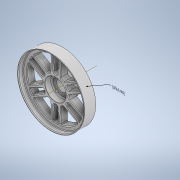
# Autodesk Inventor part: RPF1s
Saved by Autodesk Inventor 2020 (Build 240168000, 168)
## iProperties
Created: 2022-01-06
Part Number: RPF1s
Material: Generic
Document SubType Name: Modeling
Designer: harry
Density: 1 g/cm^3
Appearance: Default
Author: harry
Autodesk Inventor part; units mm, degrees
ref_plane "YZ Plane" through (0, 0, 0) normal (1, 0, 0) x (0, 1, 0)
ref_plane "XZ Plane" through (0, 0, 0) normal (0, 1, 0) x (-1, 0, 0)
ref_plane "Work Plane1" through (0, 0, 35) normal (0, 0, 1) x (1, 0, 0)
sketch "Sketch2" plane through (0, 0, 35) normal (0, 0, 1) x (1, 0, 0)
  circle A0 centre (0, 0) radius 75.361
  circle A1 centre (0, 0) radius 37.761
  circle A2 centre (-57.1499, 18.5691) radius 7.75
  circle A3 centre (0, 60.091) radius 7.75
  circle A4 centre (57.1499, 18.5691) radius 7.75
  circle A5 centre (35.3206, -48.6146) radius 7.75
  circle A6 centre (-35.3206, -48.6146) radius 7.75
  dimension "d2" = 37.6
  dimension "d3" = 150.722
  dimension "d4" = 15.5
  dimension "d7" = 360
  dimension "d11" = 60.091
  constraints: 7 centre point, 4 coincident, 1 vertical alignment, 14 other
  measures "d2" radial gap between concentric circles of A0 A1
  measures "d3" diameter of A0
  measures "d4" diameter of A2
  measures "d11" distance of A0.centre A3.centre
sketch "Sketch3" plane through (0, 0, 0) normal (1, 0, 0) x (0, 1, 0)
  line L0 (-273.6168, 35) -> (133.524, 35) construction
  line L1 (75.361, 35) -> (75.361, 71.76) construction
  line L2 (75.361, 35) -> (-75.361, 35) construction
  line L3 (75.361, 71.76) -> (75.361, 35)
  line L4 (0, -28.552) -> (0, 171.312) construction
  line L5 (75.361, 71.76) -> (0, 71.76)
  line L6 (0, 35) -> (0, 71.76)
  line L7 (0, 35) -> (75.361, 35)
  point P0 (0, 0)
  dimension "d91" = 36.76
  constraints: 10 end point, 2 collinear, 2 perpendicular, 2 point on line, 1 midpoint
  measures "d91" distance between parallel lines of L2 L5
revolve "Revolution1" add sketch "Sketch3" angle 360 about axis through (0, 0, -10) along (0, 0, 1)
extrude "Extrusion1" cut sketch "Sketch2" along normal through all contours A1 | A2 | A3 | A4 | A5 | A6
ref_plane "Work Plane2" through (0, 0, 71.76) normal (0, 0, 1) x (1, 0, 0)
sketch "Sketch4" plane through (0, 0, 71.76) normal (0, 0, 1) x (1, 0, 0)
  line L0 (-13, 95.7863) -> (-17, 184.2173)
  line L1 (-34.3721, 75.9448) -> (-32.5, 182.1229)
  circle A0 centre (0, 0) radius 185
  line L2 (13, 95.7863) -> (17, 184.2173)
  line L3 (34.3721, 75.9448) -> (32.5, 182.1229)
  arc A1 (-13, 95.7863) -> (13, 95.7863) centre (0, 96.3743) ccw
  circle A2 centre (0, 0) radius 68.5449
  circle A3 centre (0, 0) radius 83.361
  circle A4 centre (0, 0) radius 68.5449
  arc A5 (-89.4533, 36.6348) -> (-76.4533, 59.1515) centre (-83.4626, 48.1871) ccw
  line L4 (-48.5841, 67.7395) -> (-141.4731, 119.2073)
  line L5 (-76.4533, 59.1515) -> (-151.0368, 106.8311)
  line L6 (-89.4533, 36.6348) -> (-168.0368, 77.3862)
  line L7 (-82.9562, 8.2053) -> (-173.9731, 62.9156)
  arc A6 (-76.4533, -59.1515) -> (-89.4533, -36.6348) centre (-83.4626, -48.1871) ccw
  line L8 (-82.9562, -8.2053) -> (-173.9731, -62.9156)
  line L9 (-89.4533, -36.6348) -> (-168.0368, -77.3862)
  line L10 (-76.4533, -59.1515) -> (-151.0368, -106.8311)
  line L11 (-48.5841, -67.7395) -> (-141.4731, -119.2073)
  arc A7 (13, -95.7863) -> (-13, -95.7863) centre (0, -96.3743) ccw
  line L12 (-34.3721, -75.9448) -> (-32.5, -182.1229)
  line L13 (-13, -95.7863) -> (-17, -184.2173)
  line L14 (13, -95.7863) -> (17, -184.2173)
  line L15 (34.3721, -75.9448) -> (32.5, -182.1229)
  arc A8 (89.4533, -36.6348) -> (76.4533, -59.1515) centre (83.4626, -48.1871) ccw
  line L16 (48.5841, -67.7395) -> (141.4731, -119.2073)
  line L17 (76.4533, -59.1515) -> (151.0368, -106.8311)
  line L18 (89.4533, -36.6348) -> (168.0368, -77.3862)
  line L19 (82.9562, -8.2053) -> (173.9731, -62.9156)
  arc A9 (76.4533, 59.1515) -> (89.4533, 36.6348) centre (83.4626, 48.1871) ccw
  line L20 (82.9562, 8.2053) -> (173.9731, 62.9156)
  line L21 (89.4533, 36.6348) -> (168.0368, 77.3862)
  line L22 (76.4533, 59.1515) -> (151.0368, 106.8311)
  line L23 (48.5841, 67.7395) -> (141.4731, 119.2073)
  circle A10 centre (0, 0) radius 210
  arc A11 (-56.3873, 72.0631) -> (-34.2148, 84.8644) centre (-49.1485, 85.1277) ccw
  arc A12 (-90.6021, -12.8013) -> (-90.6021, 12.8013) centre (-98.297, 0) ccw
  arc A13 (-34.2148, -84.8644) -> (-56.3873, -72.0631) centre (-49.1485, -85.1277) ccw
  arc A14 (56.3873, -72.0631) -> (34.2148, -84.8644) centre (49.1485, -85.1277) ccw
  arc A15 (90.6021, 12.8013) -> (90.6021, -12.8013) centre (98.297, 0) ccw
  arc A16 (34.2148, 84.8644) -> (56.3873, 72.0631) centre (49.1485, 85.1277) ccw
  circle A17 centre (0, 0) radius 83.361 projected
  point P0 (-168.0368, 77.3862)
  point P1 (-151.0368, 106.8311)
  point P2 (-141.4731, 119.2073)
  point P3 (-17, -184.2173)
  point P4 (34.2148, -84.8644)
  point P5 (56.3873, -72.0631)
  point P6 (168.0368, 77.3862)
  point P7 (56.3873, 72.0631)
  point P8 (34.2148, 84.8644)
  point P9 (141.4731, 119.2073)
  point P10 (90.6021, -12.8013)
  point P11 (90.6021, 12.8013)
  point P12 (173.9731, 62.9156)
  point P13 (168.0368, -77.3862)
  point P14 (151.0368, -106.8311)
  point P15 (-56.3873, -72.0631)
  point P16 (-34.2148, -84.8644)
  point P17 (-141.4731, -119.2073)
  point P18 (-151.0368, -106.8311)
  point P19 (-168.0368, -77.3862)
  point P20 (-90.6021, 12.8013)
  point P21 (-90.6021, -12.8013)
  point P22 (-173.9731, -62.9156)
  point P23 (-173.9731, 62.9156)
  dimension "d43" = 3.6
  dimension "d49" = 3.6
  dimension "d50" = 26
  dimension "d51" = 34
  dimension "d54" = 65
  dimension "d57" = 370
  dimension "d61" = 360
  dimension "d63" = 25
  dimension "d66" = 360
  dimension "d83" = 137.0898
  constraints: 48 end point, 30 point on circle, 17 centre point, 6 tangent, 4 coincident, 4 concentric, 2 equal length, 2 point on line, 1 vertical alignment, 110 other
  measures "d43" angle of L0 L1
  measures "d49" angle of L3 L2
  measures "d50" distance of L2.start L0.start
  measures "d51" distance of L2.end L0.end
  measures "d54" distance of L1.end L3.end
  measures "d57" diameter of A0
  measures "d63" radial gap between concentric circles of A10 A0
  measures "d83" diameter of A2
extrude "Extrusion2" add sketch "Sketch4" along normal blind 45 contours A1 A3 L1 A0 L0 | A1 L2 A0 L3 A3 | A3 | L3 A16 A3 | A3 A11 L1 | L4 A3 A5 L5 A0 | A16 L23 A3 | A3 L4 A11 | A0 L22 A9 A3 L23 | L6 A5 A3 L7 A0 | A9 L21 A0 L20 A3 | L20 A15 A3 | A3 A12 L7 | L8 A3 A6 L9 A0 | A15 L19 A3 | A3 L8 A12 | L19 A0 L18 A8 A3 | L10 A6 A3 L11 A0 | A8 L17 A0 L16 A3 | L16 A14 A3 | A3 A13 L11 | L12 A3 A7 L13 A0 | A14 L15 A3 | A3 L12 A13 | L15 A0 L14 A7 A3 | A10
fillet "Fillet2" radius 4 24 edges at (141.4731, 119.2073, 94.26) (168.0368, 77.3862, 94.26) (-141.4731, 119.2073, 94.26) (-168.0368, 77.3862, 94.26) (-32.5, 182.1229, 94.26) (17, 184.2173, 94.26) (-151.0368, 106.8311, 94.26) (168.0368, -77.3862, 94.26) (141.4731, -119.2073, 94.26) (-141.4731, -119.2073, 94.26) (-168.0368, -77.3862, 94.26) (-17, -184.2173, 94.26) (32.5, -182.1229, 94.26) (-32.5, -182.1229, 94.26) (17, -184.2173, 94.26) (151.0368, -106.8311, 94.26) (173.9731, -62.9156, 94.26) (-151.0368, -106.8311, 94.26) (-173.9731, -62.9156, 94.26) (-173.9731, 62.9156, 94.26) (32.5, 182.1229, 94.26) (-17, 184.2173, 94.26) (151.0368, 106.8311, 94.26) (173.9731, 62.9156, 94.26)
fillet "Fillet3" radius 4.6 72 edges at (34.0326, 180.3425, 116.76) (92.5, 160.2147, 116.76) (139.1649, 119.6444, 116.76) (96.7739, 94.4404, 116.76) (41.6805, 72.1927, 116.76) (33.4009, 131.0288, 116.76) (0, 83.361, 116.76) (-14.9129, 138.0751, 116.76) (-15.8176, 183.2042, 116.76) (0, 185, 116.76) (15.8176, 183.2042, 116.76) (14.9129, 138.0751, 116.76) (-139.1649, 119.6444, 116.76) (-92.5, 160.2147, 116.76) (-34.0326, 180.3425, 116.76) (-33.4009, 131.0288, 116.76) (-41.6805, 72.1927, 116.76) (-96.7739, 94.4404, 116.76) (-166.5683, 77.9037, 116.76) (-160.2147, 92.5, 116.76) (-150.7507, 105.3006, 116.76) (-112.1201, 81.9525, 116.76) (-72.1927, 41.6805, 116.76) (-127.033, 56.1227, 116.76) (-83.361, 0, 116.76) (-130.1747, -36.5884, 116.76) (-173.1975, -60.6982, 116.76) (-185, 0, 116.76) (-173.1975, 60.6982, 116.76) (-130.1747, 36.5884, 116.76) (-150.7507, -105.3006, 116.76) (-160.2147, -92.5, 116.76) (-166.5683, -77.9037, 116.76) (-127.033, -56.1227, 116.76) (-72.1927, -41.6805, 116.76) (-112.1201, -81.9525, 116.76) (-41.6805, -72.1927, 116.76) (-33.4009, -131.0288, 116.76) (-34.0326, -180.3425, 116.76) (-92.5, -160.2147, 116.76) (-139.1649, -119.6444, 116.76) (-96.7739, -94.4404, 116.76) (14.9129, -138.0751, 116.76) (15.8176, -183.2042, 116.76) (0, -185, 116.76) (-15.8176, -183.2042, 116.76) (-14.9129, -138.0751, 116.76) (0, -83.361, 116.76) (139.1649, -119.6444, 116.76) (92.5, -160.2147, 116.76) (34.0326, -180.3425, 116.76) (33.4009, -131.0288, 116.76) (41.6805, -72.1927, 116.76) (96.7739, -94.4404, 116.76) (166.5683, -77.9037, 116.76) (160.2147, -92.5, 116.76) (150.7507, -105.3006, 116.76) (112.1201, -81.9525, 116.76) (72.1927, -41.6805, 116.76) (127.033, -56.1227, 116.76) (83.361, 0, 116.76) (130.1747, 36.5884, 116.76) (173.1975, 60.6982, 116.76) (185, 0, 116.76) (173.1975, -60.6982, 116.76) (130.1747, -36.5884, 116.76) (72.1927, 41.6805, 116.76) (112.1201, 81.9525, 116.76) (150.7507, 105.3006, 116.76) (160.2147, 92.5, 116.76) (166.5683, 77.9037, 116.76) (127.033, 56.1227, 116.76)
fillet "Fillet1" radius 1.5 1 edges at (-68.5449, 0, 116.76)
sketch "Sketch5" plane through (0, 0, 0) normal (1, 0, 0) x (0, 1, 0)
  line L0 (210, 116.76) -> (-210, 116.76) projected
  line L1 (-210, 116.76) -> (-210.4538, 142.76)
  line L2 (-210.4538, 142.76) -> (-215.4538, 142.76)
  line L3 (-215.4538, 142.76) -> (-215.4538, 71.76)
  line L4 (210, 71.76) -> (-210, 71.76) projected
  line L5 (-215.4538, 71.76) -> (-210, 71.76)
  line L6 (-210, 116.76) -> (-210, 71.76)
  line L7 (0, -29.9756) -> (0, 179.8535) projected
  arc A0 (-215.4538, 142.76) -> (-216.8172, 147.5225) centre (-224.4538, 142.76) ccw
  line L8 (-216.8172, 147.5225) -> (-213.6324, 147.5225)
  arc A1 (-213.6324, 147.5225) -> (-210.4538, 142.76) centre (-204.9461, 149.8779) ccw
  dimension "d77" = 91
  dimension "d78" = 5
  dimension "d79" = 26
  dimension "d85" = 9
  dimension "d86" = 4.7625
  constraints: 12 end point, 4 point on circle, 3 horizontal, 2 centre point, 1 equal radius, 1 perpendicular, 1 tangent, 1 vertical
  measures "d77" angle of L0 L1
  measures "d78" distance of L1.end L2.end
  measures "d79" distance between parallel lines of L2 L0
  measures "d85" radius of A0
  measures "d86" distance between parallel lines of L8 L2
revolve "Revolution2" add sketch "Sketch5" angle 360 about axis through (0, 0, -10) along (0, 0, 1) contours L6 L5 L3 L2 L1 | L2 A0 L8 A1
fillet "Fillet5" radius 4 1 edges at (0, 210, 116.76)
sketch "Sketch7" plane through (0, 0, 0) normal (1, 0, 0) x (0, 1, 0)
  line L0 (83.361, 71.76) -> (95.7863, 71.76) projected
  line L1 (-75.361, 35) -> (75.361, 35) projected
  arc A0 (83.361, 71.76) -> (75.361, 35) centre (163.8171, 35) ccw
  line L2 (-75.361, 71.76) -> (75.361, 71.76) projected
  line L3 (83.361, 71.76) -> (75.361, 71.76)
  line L4 (75.361, 71.76) -> (75.361, 35)
  line L5 (0, -29.5045) -> (0, 177.027) projected
  point P0 (0, 0)
  constraints: 4 end point, 2 point on circle, 1 centre point, 1 collinear, 1 horizontal alignment, 1 perpendicular
revolve "Revolution3" add sketch "Sketch7" angle 360 about axis through (0, 0, -10) along (0, 0, 1) contours L4 L3 A0
fillet "Fillet6" radius 8 1 edges at (-68.5449, 0, 71.76)
body "Solid1"
